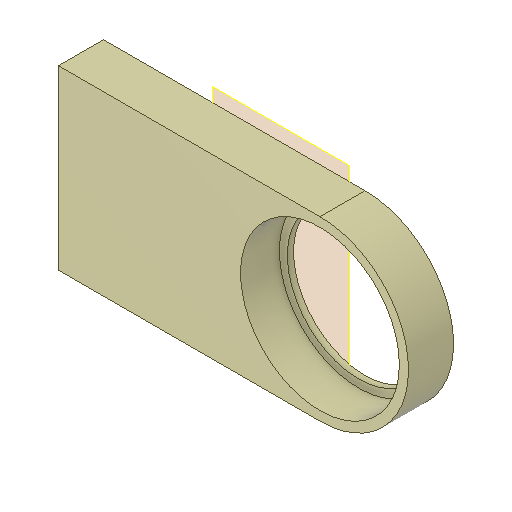
# Autodesk Inventor part: 00_Filteslide_25mm_sandwich
Saved by Autodesk Inventor 2022.5 (Build 265521000, 521)
## iProperties
Created: 2019-08-26
Part Number: 00_Filteslide_25mm_sandwich
Material: Generic
Document SubType Name: Modeling
Designer: diederichbenedict
Density: 1 g/cm^3
Appearance: Smooth - Ash
Author: diederichbenedict
Autodesk Inventor part; units mm, degrees
ref_plane "YZ Plane" through (0, 0, 0) normal (1, 0, 0) x (0, 1, 0)
ref_plane "XZ Plane" through (0, 0, 0) normal (0, 1, 0) x (-1, 0, 0)
ref_plane "XY Plane" through (0, 0, 0) normal (0, 0, 1) x (1, 0, 0)
ref_plane "Work Plane1" through (0, 0, 0) normal (0, 0, 1) x (1, 0, 0)
sketch "Sketch1" plane through (0, 0, 0) normal (0, 0, 1) x (1, 0, 0)
  arc A0 (-18.155, 30) -> (-18.155, 0) centre (0, 15) ccw construction
  line L0 (-18.155, 0) -> (-3.4871, 0) construction
  line L1 (-18.155, 30) -> (-3.4871, 30) construction
  circle A1 centre (0, 15) radius 15.4 construction
  arc A2 (-6.5238, 29.25) -> (-6.5238, 0.75) centre (0, 15) ccw construction
  line L2 (-6.5238, 0.75) -> (-17.7982, 0.75) construction
  arc A3 (-17.7982, 29.25) -> (-17.7982, 0.75) centre (0, 15) ccw construction
  line L3 (-17.7982, 29.25) -> (-6.5238, 29.25) construction
  circle A4 centre (0, 15) radius 12.775 construction
  line L4 (-6.5238, 29.25) -> (0, 29.25) construction
  line L5 (-6.5238, 0.75) -> (0, 0.75) construction
  arc A5 (0, 0.75) -> (0, 29.25) centre (0, 15) ccw construction
  line L6 (-42.0841, 29.25) -> (-42.0841, 0.75)
  line L7 (-42.0841, 0.75) -> (0, 0.75)
  line L8 (-42.0841, 29.25) -> (0, 29.25)
  circle A6 centre (0, 15) radius 11.5
  arc A7 (0, 0.75) -> (0, 29.25) centre (0, 15) ccw
  arc A8 (-3.4871, 0) -> (3.4871, 0) centre (0, 15) ccw projected
  line L9 (3.4871, 0) -> (18, 0) projected
  line L10 (18, 0) -> (18, 30) projected
  line L11 (3.4871, 30) -> (18, 30) projected
  arc A9 (3.4871, 30) -> (-3.4871, 30) centre (0, 15) ccw projected
  line L12 (-7.3927, 28.5095) -> (7.3927, 28.5095) projected
  arc A10 (7.3927, 1.4905) -> (7.3927, 28.5095) centre (0, 15) ccw projected
  line L13 (7.3927, 1.4905) -> (-7.3927, 1.4905) projected
  arc A11 (-7.3927, 28.5095) -> (-7.3927, 1.4905) centre (0, 15) ccw projected
  point P0 (0, 0)
  dimension "d0" = 0.75
  dimension "d1" = 25.55
  dimension "d2" = 23
  constraints: 14 end point, 8 point on circle, 6 centre point, 3 tangent, 2 coincident, 2 point on line, 1 parallel, 1 perpendicular, 1 vertical, 2 other
  measures "d0" distance between parallel lines of L1 L3
  measures "d1" diameter of A4
  measures "d2" diameter of A6
extrude "Extrusion1" add sketch "Sketch1" along normal blind 1 contours L8 A7 L12 A11 L13 L7 L6 | A7 L13 A11 L12
sketch "Sketch2" plane through (0, 0, 1) normal (0, 0, 1) x (1, 0, 0)
  circle A0 centre (0, 15) radius 11.5 projected
  line L0 (0, 29.25) -> (-42.0841, 29.25) projected
  line L1 (-42.0841, 29.25) -> (-42.0841, 0.75) projected
  line L2 (-42.0841, 0.75) -> (0, 0.75) projected
  arc A1 (0, 0.75) -> (0, 29.25) centre (0, 15) ccw projected
  circle A2 centre (0, 15) radius 12.775
  point P0 (0, 0)
  dimension "d5" = 25.55
  constraints: 1 centre point, 1 coincident
  measures "d5" diameter of A2
extrude "Extrusion2" add sketch "Sketch2" along normal blind 6.25 contours A1 L2 L1 L0
body "Solid1"
